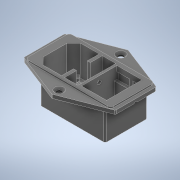
# Autodesk Inventor part: AC-14-F16A
Saved by Autodesk Inventor 2021 (Build 250183000, 183)
## iProperties
Created: 2021-04-10
Part Number: AC-14-F16A
Material: Generic
Document SubType Name: Modeling
Designer: Andrew
Density: 1 g/cm^3
Appearance: Smooth - Black
Author: Andrew
Autodesk Inventor part; units mm, degrees
ref_plane "YZ Plane" through (0, 0, 0) normal (1, 0, 0) x (0, 1, 0)
ref_plane "XZ Plane" through (0, 0, 0) normal (0, 1, 0) x (-1, 0, 0)
ref_plane "XY Plane" through (0, 0, 0) normal (0, 0, 1) x (1, 0, 0)
sketch "Sketch1" plane through (0, 0, 0) normal (0, 1, 0) x (-1, 0, 0)
  line L0 (27.65, 0) -> (-27.65, 0)
  line L1 (-27.65, 0) -> (-27.65, -12.25)
  line L2 (-25.65, -14.25) -> (25.65, -14.25)
  line L3 (27.65, -12.25) -> (27.65, 0)
  line L4 (29.75, 0) -> (-29.75, 0)
  line L5 (-29.75, 0) -> (-29.75, -12.5644)
  line L6 (29.75, -12.5644) -> (29.75, 0)
  line L7 (29.1106, -13.4972) -> (0.3606, -24.6106)
  line L8 (-0.3606, -24.6106) -> (-29.1106, -13.4972)
  arc A0 (-27.65, -12.25) -> (-25.65, -14.25) centre (-25.65, -12.25) ccw
  arc A1 (25.65, -14.25) -> (27.65, -12.25) centre (25.65, -12.25) ccw
  arc A2 (-29.75, -12.5644) -> (-29.1106, -13.4972) centre (-28.75, -12.5644) ccw
  arc A3 (29.1106, -13.4972) -> (29.75, -12.5644) centre (28.75, -12.5644) ccw
  arc A4 (-0.3606, -24.6106) -> (0.3606, -24.6106) centre (0, -23.6779) ccw
  line L9 (23.625, -8.125) -> (23.625, 0)
  line L10 (23.625, 0) -> (-23.625, 0)
  line L11 (-23.625, 0) -> (-23.625, -12.75)
  line L12 (-22.625, -13.75) -> (18, -13.75)
  line L13 (18, -13.75) -> (23.625, -8.125)
  arc A5 (-23.625, -12.75) -> (-22.625, -13.75) centre (-22.625, -12.75) ccw
  point P0 (0, 0)
  point P1 (-27.65, -14.25)
  point P2 (27.65, -14.25)
  point P3 (-29.75, -13.25)
  point P4 (29.75, -13.25)
  point P5 (0, -24.75)
  point P6 (0, 0)
  point P7 (0, -20)
  point P8 (23.625, 0)
  dimension "d0" = 59.5
  dimension "d1" = 55.3
  dimension "d2" = 14.25
  dimension "d3" = 13.25
  dimension "d4" = 24.75
  dimension "d5" = 2
  dimension "d6" = 1
  dimension "d7" = 1
  dimension "d12" = 20
  dimension "d18" = 13.75
  dimension "d19" = 47.25
  dimension "d20" = 45
  dimension "d21" = 8.125
  dimension "d22" = 1
  constraints: 28 end point, 13 point on line, 12 point on circle, 12 tangent, 6 centre point, 4 perpendicular, 3 midpoint, 3 parallel, 2 equal radius, 2 horizontal, 1 coincident, 1 horizontal alignment, 1 vertical, 1 vertical alignment
  measures "d0" distance between parallel lines of L5 L6
  measures "d1" distance of point (-27.65, -14.25) point (27.65, -14.25)
  measures "d2" distance of L0.end point (-27.65, -14.25)
  measures "d3" distance of L4.end point (-29.75, -13.25)
  measures "d4" distance from line of L0 point (0, -24.75)
  measures "d5" radius of A0
  measures "d6" radius of A2
  measures "d7" radius of A4
  measures "d12" distance from line of L4 point (0, -20)
  measures "d18" distance between parallel lines of L4 L12
  measures "d19" distance between parallel lines of L11 L9
  measures "d20" angle of L12 L13
  measures "d21" distance of L9.start L9.end
  measures "d22" radius of A5
extrude "Extrusion1" add sketch "Sketch1" along normal blind 2.35 contours L4 L6 A3 L7 A4 L8 A2 L5 L1 A0 L2 A1 L3
extrude "Extrusion2" add sketch "Sketch1" along normal blind 3.35 contours L3 A1 L2 A0 L1 L0 L11 A5 L12 L13 L9 | L9 L13 L12 A5 L11 L0
sketch "Sketch2" plane through (0, 0, 0) normal (1, 0, 0) x (0, 1, 0)
  line L0 (0, -20) -> (2.35, -20)
  line L1 (2.35, -20) -> (2.35, -23)
  line L2 (2.35, -23) -> (1.1, -21.75)
  line L3 (1.1, -21.75) -> (0, -21.75)
  line L4 (2.35, -14.25) -> (2.35, -12.25) projected
  line L5 (2.35, -12.25) -> (2.35, 0) projected
  line L6 (2.35, 0) -> (2.35, -12.5644) projected
  line L7 (2.35, -12.5644) -> (2.35, -13.4972) projected
  line L8 (2.35, -13.4972) -> (2.35, -24.6106) construction
  line L9 (2.35, -24.6106) -> (2.35, -24.6106) projected
  line L10 (2.35, -24.6106) -> (2.35, -13.4972) projected
  line L11 (2.35, -13.4972) -> (2.35, -12.5644) projected
  line L12 (2.35, -12.5644) -> (2.35, 0) projected
  line L13 (2.35, 0) -> (2.35, -12.25) projected
  line L14 (2.35, -12.25) -> (2.35, -14.25) projected
  line L15 (0, -20) -> (0, -21.75)
  point P0 (0, 0)
  dimension "d13" = 3
  dimension "d14" = 1.75
  dimension "d16" = 45
  constraints: 10 end point, 1 collinear, 1 horizontal, 1 parallel, 1 perpendicular, 1 vertical
  measures "d13" distance of L0.end L1.end
  measures "d14" distance between parallel lines of L0 L3
  measures "d16" angle of L2 L1
revolve "Revolution1" cut sketch "Sketch2" angle 360 about axis through (0, 0, -20) along (0, 1, 0)
extrude "Extrusion3" add sketch "Sketch1" against normal blind 18.75 contours L9 L13 L12 A5 L11 L0
mirror "Mirror1" about plane through (0, 0, 0) normal (0, 0, 1)
sketch "Sketch3" plane through (0, 0, 0) normal (0, 1, 0) x (-1, 0, 0)
  line L0 (22.75, 0) -> (22.75, -7.75)
  line L1 (22.75, -7.75) -> (18.25, -12.25)
  line L2 (18.25, -12.25) -> (6.25, -12.25)
  line L3 (6.25, -12.25) -> (6.25, -4.5)
  line L4 (6.25, -4.5) -> (4.25, -4.5)
  line L5 (4.25, -4.5) -> (4.25, -12.25)
  line L6 (4.25, -12.25) -> (-4.5, -12.25)
  line L7 (-4.5, -12.25) -> (-4.5, 0)
  line L8 (-4.5, 0) -> (22.75, 0)
  line L9 (-6, 0) -> (-22.25, 0)
  line L10 (-22.25, 0) -> (-22.25, -11.5)
  line L11 (-22.25, -11.5) -> (-6, -11.5)
  line L12 (-6, -11.5) -> (-6, 0)
  line L13 (29.75, 0) -> (-29.75, 0) construction
  line L14 (-6, -9.625) -> (-22.25, -9.625)
  line L15 (-13.75, 0) -> (-14.5, 0)
  line L16 (-14.5, 0) -> (-14.5, -9.625)
  line L17 (-14.5, -9.625) -> (-13.75, -9.625)
  line L18 (-13.75, -9.625) -> (-13.75, 0)
  line L19 (-13.125, 0) -> (-15.125, 0)
  line L20 (-15.125, 0) -> (-15.125, -2)
  line L21 (-15.125, -2) -> (-13.125, -2)
  line L22 (-13.125, -2) -> (-13.125, 0)
  line L23 (-6.875, -5.125) -> (-12.875, -5.125)
  line L24 (-12.875, -5.125) -> (-12.875, -5.625)
  line L25 (-12.875, -5.625) -> (-6.875, -5.625)
  line L26 (-6.875, -5.625) -> (-6.875, -5.125)
  line L27 (-15.375, -9.125) -> (-21.375, -9.125)
  line L28 (-21.375, -9.125) -> (-21.375, -9.625)
  line L29 (-21.375, -9.625) -> (-15.375, -9.625)
  line L30 (-15.375, -9.625) -> (-15.375, -9.125)
  line L31 (-6.875, 0) -> (-12.875, 0)
  line L32 (-12.875, 0) -> (-12.875, -0.25)
  line L33 (-12.875, -0.25) -> (-6.875, -0.25)
  line L34 (-6.875, -0.25) -> (-6.875, 0)
  line L35 (-9.875, 0) -> (-9.875, -5.125) construction
  line L36 (-18.375, -9.125) -> (-18.375, 0) construction
  line L37 (-6, -11.5) -> (-6, -13)
  line L38 (-6, -13) -> (-22.25, -13)
  line L39 (-22.25, -13) -> (-22.25, -11.5)
  line L40 (-14.25, -11.5) -> (-14.25, -13)
  line L41 (-16.25, -11.5) -> (-16.25, -13)
  line L42 (-6, 0) -> (-13.75, 0)
  line L43 (-13.75, 0) -> (-13.75, -0.25)
  line L44 (-13.75, -0.25) -> (-6, -0.25)
  line L45 (-6, -0.25) -> (-6, 0)
  line L46 (-6, -5.125) -> (-13.75, -5.125)
  line L47 (-13.75, -5.125) -> (-13.75, -5.625)
  line L48 (-13.75, -5.625) -> (-6, -5.625)
  line L49 (-6, -5.625) -> (-6, -5.125)
  line L50 (-14.5, -9.125) -> (-22.25, -9.125)
  line L51 (-22.25, -9.125) -> (-22.25, -9.625)
  line L52 (-22.25, -9.625) -> (-14.5, -9.625)
  line L53 (-14.5, -9.625) -> (-14.5, -9.125)
  line L54 (-14.5, 0) -> (-22.25, 0)
  line L55 (-22.25, 0) -> (-22.25, -0.25)
  line L56 (-22.25, -0.25) -> (-14.5, -0.25)
  line L57 (-14.5, -0.25) -> (-14.5, 0)
  line L58 (-15.375, 0) -> (-21.375, 0)
  line L59 (-21.375, 0) -> (-21.375, -0.25)
  line L60 (-21.375, -0.25) -> (-15.375, -0.25)
  line L61 (-15.375, -0.25) -> (-15.375, 0)
  line L62 (-16.25, -12.25) -> (-22.25, -12.25)
  line L63 (-14.25, -12.25) -> (-6, -12.25)
  line L64 (-6, 0) -> (-6.625, 0)
  line L65 (-6.625, 0) -> (-6.625, -2)
  line L66 (-6.625, -2) -> (-6, -2)
  line L67 (-6, -2) -> (-6, 0)
  line L68 (-22.25, 0) -> (-21.625, 0)
  line L69 (-21.625, 0) -> (-21.625, -2)
  line L70 (-21.625, -2) -> (-22.25, -2)
  line L71 (-22.25, -2) -> (-22.25, 0)
  line L72 (-17.125, -9.125) -> (-19.625, -9.125)
  line L73 (-19.625, -9.125) -> (-19.625, -5.625)
  line L74 (-19.625, -5.625) -> (-17.125, -5.625)
  line L75 (-17.125, -5.625) -> (-17.125, -9.125)
  line L76 (-8.625, -5.625) -> (-11.125, -5.625)
  line L77 (-11.125, -5.625) -> (-11.125, -9.125)
  line L78 (-11.125, -9.125) -> (-8.625, -9.125)
  line L79 (-8.625, -9.125) -> (-8.625, -5.625)
  line L80 (-8.625, 0) -> (-11.125, 0)
  line L81 (-11.125, 0) -> (-11.125, -1.5)
  line L82 (-11.125, -1.5) -> (-8.625, -1.5)
  line L83 (-8.625, -1.5) -> (-8.625, 0)
  line L84 (-17.125, 0) -> (-19.625, 0)
  line L85 (-19.625, 0) -> (-19.625, -1.5)
  line L86 (-19.625, -1.5) -> (-17.125, -1.5)
  line L87 (-17.125, -1.5) -> (-17.125, 0)
  line L88 (16.25, -9) -> (8.25, -9)
  line L89 (8.25, -9) -> (8.25, -5)
  line L90 (8.25, -5) -> (16.25, -5)
  line L91 (16.25, -5) -> (16.25, -9)
  line L92 (16.25, -8.25) -> (8.25, -8.25)
  line L93 (8.25, -8.25) -> (8.25, -5.75)
  line L94 (8.25, -5.75) -> (16.25, -5.75)
  line L95 (16.25, -5.75) -> (16.25, -8.25)
  line L96 (20.75, 0) -> (12.75, 0)
  line L97 (12.75, 0) -> (12.75, -2)
  line L98 (12.75, -2) -> (20.75, -2)
  line L99 (20.75, -2) -> (20.75, 0)
  line L100 (14.75, -8.25) -> (9.75, -8.25)
  line L101 (9.75, -8.25) -> (9.75, -5.75)
  line L102 (9.75, -5.75) -> (14.75, -5.75)
  line L103 (14.75, -5.75) -> (14.75, -8.25)
  line L104 (20.25, 0) -> (13.25, 0)
  line L105 (13.25, 0) -> (13.25, -1.25)
  line L106 (13.25, -1.25) -> (20.25, -1.25)
  line L107 (20.25, -1.25) -> (20.25, 0)
  line L108 (18.6036, -11.8964) -> (20.0178, -10.4822)
  line L109 (20.0178, -10.4822) -> (18.6036, -9.068)
  line L110 (18.6036, -9.068) -> (17.1893, -10.4822) construction
  line L111 (17.1893, -10.4822) -> (18.6036, -11.8964)
  arc A0 (18.6036, -9.068) -> (17.1893, -10.4822) centre (17.8964, -9.7751) ccw
  point P0 (0, 0)
  point P1 (-14.125, 0)
  point P2 (-6.625, 0)
  point P3 (-9.875, -5.625)
  point P4 (-9.875, 0)
  point P5 (-18.375, 0)
  point P6 (-8.625, -0.25)
  point P7 (-11.125, -0.25)
  point P8 (-17.125, -0.25)
  point P9 (-19.625, -0.25)
  point P10 (12.25, -8.25)
  point P11 (16.75, 0)
  dimension "d25" = 11.5
  dimension "d26" = 16.25
  dimension "d27" = 7.5
  dimension "d28" = 1.5
  dimension "d29" = 2
  dimension "d30" = 8.75
  dimension "d31" = 12.25
  dimension "d32" = 4.5
  dimension "d33" = 45
  dimension "d34" = 7
  dimension "d35" = 7.75
  dimension "d40" = 9.625
  dimension "d43" = 0.75
  dimension "d44" = 6
  dimension "d45" = 6
  dimension "d46" = 0.5
  dimension "d47" = 0.25
  dimension "d48" = 0.5
  dimension "d49" = 4
  dimension "d50" = 2
  dimension "d51" = 2
  dimension "d52" = 1.5
  dimension "d53" = 2
  dimension "d54" = 6
  dimension "d61" = 0.625
  dimension "d62" = 0.625
  dimension "d71" = 2.5
  dimension "d72" = 2.5
  dimension "d73" = 1.5
  dimension "d81" = 8
  dimension "d82" = 8
  dimension "d83" = 0.75
  dimension "d84" = 0.75
  dimension "d85" = 5
  dimension "d86" = 2.5
  dimension "d87" = 4
  dimension "d88" = 6
  dimension "d89" = 6
  dimension "d90" = 7
  dimension "d91" = 1.25
  dimension "d92" = 2
  dimension "d93" = 2
  dimension "d94" = 2
  dimension "d95" = 0.5
  constraints: 222 end point, 46 parallel, 34 perpendicular, 32 point on line, 23 horizontal, 22 midpoint, 14 collinear, 2 point on circle, 2 tangent, 2 vertical, 1 centre point, 8 other
  measures "d25" distance of L9.end L10.end
  measures "d26" distance of L10.end L11.end
  measures "d27" distance from line of point (-29.75, 0) L10
  measures "d28" distance between parallel lines of L12 L7
  measures "d29" distance of L3.end L4.end
  measures "d30" distance of L5.end L6.end
  measures "d31" distance of L6.end L7.end
  measures "d32" distance between parallel lines of L8 L4
  measures "d33" angle of L2 L1
  measures "d34" distance from line of point (29.75, 0) L0
  measures "d35" distance of L0.start L0.end
  measures "d40" distance of the line from the sketch origin of L14
  measures "d43" distance between parallel lines of L16 L18
  measures "d44" distance of L24.end L25.end
  measures "d45" distance of L28.end L29.end
  measures "d46" distance of L25.end L23.start
  measures "d47" distance of the line from the sketch origin of L33
  measures "d48" distance of L29.end L27.start
  measures "d49" distance between parallel lines of L23 L27
  measures "d50" distance between parallel lines of L20 L22
  measures "d51" distance of L21.end L19.start
  measures "d52" distance of L11.end L37.end
  measures "d53" distance between parallel lines of L41 L40
  measures "d54" distance between parallel lines of L39 L41
  measures "d61" distance between parallel lines of L10 L69
  measures "d62" distance between parallel lines of L12 L65
  measures "d71" distance between parallel lines of L77 L79
  measures "d72" distance of L73.end L74.end
  measures "d73" distance of L82.end L80.start
  measures "d81" distance of L97.end L98.end
  measures "d82" distance of L88.start L88.end
  measures "d83" distance between parallel lines of L100 L88
  measures "d84" distance between parallel lines of L90 L102
  measures "d85" distance of L100.start L100.end
  measures "d86" distance of L100.end L101.end
  measures "d87" distance between parallel lines of L2 L100
  measures "d88" distance from line of L3 point (12.25, -8.25)
  measures "d89" distance from line of L0 point (16.75, 0)
  measures "d90" distance of L105.end L106.end
  measures "d91" distance of L104.end L105.end
  measures "d92" distance of L96.end L97.end
  measures "d93" distance between parallel lines of L1 L110
  measures "d94" distance of L108.start L108.end
  measures "d95" distance from line of L1.end L111
extrude "Extrusion4" add sketch "Sketch3" against normal blind 19.75 from surface at 3.35 separate body contours L0 L1 L109 A0 L111 L2 L3 L4 L5 L6 L7 L8 L97 L98 L99 | L99 L98 L97 L8 L105 L106 L107 | L1 L111 A0 L109 | L107 L106 L105 L8 | L88 L89 L92 L91 | L92 L103 L94 L91 | L89 L94 L101 L92 | L94 L89 L90 L91 | L92 L101 L94 L103
extrude "Extrusion15" add sketch "Sketch3" against normal mid plane 10 from surface at -16.4 contours L107 L106 L105 L8 | L92 L101 L94 L103 bodies 2
extrude "Extrusion16" cut sketch "Sketch3" along normal blind 1 from surface at -16.4 contours L99 L98 L97 L8 L105 L106 L107 | L88 L89 L92 L91 | L94 L89 L90 L91 bodies 2
extrude "Extrusion17" cut sketch "Sketch3" along normal blind 0.5 from surface at -16.4 contours L92 L103 L94 L91 | L89 L94 L101 L92 bodies 2
extrude "Extrusion18" cut sketch "Sketch3" along normal blind 2 from surface at -16.4 contours L1 L111 A0 L109 bodies 2
extrude "Extrusion5" add sketch "Sketch3" against normal blind 19.25 from surface at 3.35 contours L12 L44 L65 L9 | L65 L44 L34 L9 | L12 L66 L65 L44 | L34 L33 L83 L9 | L65 L66 L12 L46 L23 L18 L21 L22 L44 L33 L81 L82 L83 | L83 L33 L81 L9 | L12 L48 L26 L46 | L81 L33 L32 L9 | L83 L82 L81 L33 | L12 L14 L18 L48 L25 L77 L78 L79 | L26 L25 L24 L23 | L32 L44 L22 L9 | L12 L11 L10 L14 | L24 L48 L18 L46 | L22 L44 L18 L9 | L14 L16 L21 L18 | L79 L78 L77 L25 | L18 L21 L16 L9 | L22 L21 L18 L44 | L14 L30 L50 L16 | L16 L56 L20 L9 | L14 L28 L27 L30 | L50 L27 L75 L74 L73 L10 L70 L69 L56 L85 L86 L87 L20 L21 L16 | L21 L20 L56 L16 | L20 L56 L61 L9 | L14 L10 L50 L28 | L61 L56 L87 L9 | L27 L73 L74 L75 | L87 L56 L85 L9 | L85 L56 L59 L9 | L87 L86 L85 L56 | L10 L56 L69 L70 | L59 L56 L69 L9 | L10 L9 L69 L56 bodies 2
extrude "Extrusion6" cut sketch "Sketch3" along normal blind 11.5 from surface at -15.9 contours L12 L11 L10 L14 bodies 2
extrude "Extrusion7" add sketch "Sketch3" along normal blind 5 from surface at -18.75 contours L37 L63 L40 L11 | L37 L38 L40 L63 | L41 L62 L39 L11 | L41 L38 L39 L62 bodies 2
extrude "Extrusion8" add sketch "Sketch3" along normal blind 18.6 from surface at -18.75 contours L37 L63 L40 L11 | L41 L62 L39 L11 bodies 2
extrude "Extrusion9" add sketch "Sketch3" along normal blind 1.75 from surface at -18.75 contours L40 L38 L41 L11 bodies 2
extrude "Extrusion10" cut sketch "Sketch3" along normal blind 1.75 from surface at -15.9 contours L12 L44 L65 L9 | L12 L66 L65 L44 | L22 L44 L18 L9 | L18 L21 L16 L9 | L22 L21 L18 L44 | L16 L56 L20 L9 | L21 L20 L56 L16 | L10 L56 L69 L70 | L10 L9 L69 L56 bodies 2
extrude "Extrusion11" add sketch "Sketch3" along normal blind 1.75 and the other way blind 0.5 from surface at -15.9 contours L12 L44 L65 L9 | L65 L44 L34 L9 | L34 L33 L83 L9 | L83 L33 L81 L9 | L12 L48 L26 L46 | L81 L33 L32 L9 | L83 L82 L81 L33 | L26 L25 L24 L23 | L32 L44 L22 L9 | L24 L48 L18 L46 | L22 L44 L18 L9 | L79 L78 L77 L25 | L14 L30 L50 L16 | L16 L56 L20 L9 | L14 L28 L27 L30 | L20 L56 L61 L9 | L14 L10 L50 L28 | L61 L56 L87 L9 | L27 L73 L74 L75 | L87 L56 L85 L9 | L85 L56 L59 L9 | L87 L86 L85 L56 | L59 L56 L69 L9 | L10 L9 L69 L56 bodies 2
extrude "Extrusion12" cut sketch "Sketch3" along normal blind 4.5 from surface at -15.9 contours L14 L16 L21 L18 | L18 L21 L16 L9 bodies 2
extrude "Extrusion13" add sketch "Sketch3" against normal up to surface (18.75 mm away) contours L34 L33 L83 L9 | L83 L33 L81 L9 | L81 L33 L32 L9 | L26 L25 L24 L23 | L14 L28 L27 L30 | L61 L56 L87 L9 | L87 L56 L85 L9 | L85 L56 L59 L9 bodies 2
mirror "Mirror2" about plane through (0, 0, 0) normal (0, 0, 1) bodies 2
combine bodies "Combine1" operation type subtract main body 1 bodies to subtract 2
sketch "Sketch4" plane through (23.625, -18.75, -12.75) normal (1, 0, 0) x (0, 0, -1)
  circle A0 centre (-12.75, 18.25) radius 1.25
  line L0 (-0.1856, 18.75) -> (-25.3144, 18.75) projected
  point P0 (-12.75, 18.75)
  dimension "d77" = 2.5
  dimension "d78" = 0.5
  constraints: 1 centre point
  measures "d77" diameter of A0
  measures "d78" distance from line of L0 A0.centre
extrude "Extrusion14" cut sketch "Sketch4" against normal up to surface (25.25 mm away) from surface at 6.125 bodies 1
body "Solid1"
